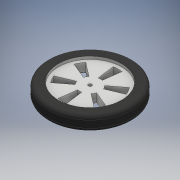
# Autodesk Inventor part: 12 in Wheel
Saved by Autodesk Inventor 2017 (Build 210142000, 142)
## iProperties
Created: 2019-11-18
Part Number: 12 in Wheel
Material: Generic
Document SubType Name: Modeling
Designer: Dell
Density: 1 g/cm^3
Appearance: Default
Author: Dell
Autodesk Inventor part; units mm, degrees
ref_plane "YZ Plane" through (0, 0, 0) normal (1, 0, 0) x (0, 1, 0)
ref_plane "XZ Plane" through (0, 0, 0) normal (0, 1, 0) x (-1, 0, 0)
ref_plane "XY Plane" through (0, 0, 0) normal (0, 0, 1) x (1, 0, 0)
sketch "Sketch1" plane through (0, 0, 0) normal (0, 0, 1) x (1, 0, 0)
  circle A0 centre (0, 0) radius 152.4
  circle A1 centre (0, 0) radius 6.35
  dimension "d0" = 304.8
  dimension "d1" = 12.7
  constraints: 2 centre point, 2 coincident
  measures "d0" diameter of A0
  measures "d1" diameter of A1
extrude "Extrusion1" add sketch "Sketch1" along normal blind 50.8
sketch "Sketch2" plane through (0, 0, 50.8) normal (0, 0, 1) x (1, 0, 0)
  circle A0 centre (0, 0) radius 6.35 projected
  circle A1 centre (0, 0) radius 38.1 construction
  circle A2 centre (0, 0) radius 101.6 construction
  line L0 (7.5, -37.3545) -> (15.7954, -100.3647)
  line L1 (-7.5, -37.3545) -> (-15.7954, -100.3647)
  line L2 (7.5, -37.3545) -> (-7.5, -37.3545) construction
  arc A3 (-15.7954, -100.3647) -> (15.7954, -100.3647) centre (0, 0) ccw
  arc A4 (-7.5, -37.3545) -> (7.5, -37.3545) centre (0, 0) ccw
  circle A5 centre (0, 0) radius 38.1 construction
  circle A6 centre (0, 0) radius 101.6 construction
  line L3 (36.1, -12.1821) -> (94.8161, -36.5031)
  line L4 (28.6, -25.1724) -> (79.0206, -63.8616)
  line L5 (36.1, -12.1821) -> (28.6, -25.1724) construction
  arc A7 (79.0206, -63.8616) -> (94.8161, -36.5031) centre (0, 0) ccw
  arc A8 (28.6, -25.1724) -> (36.1, -12.1821) centre (0, 0) ccw
  circle A9 centre (0, 0) radius 38.1 construction
  circle A10 centre (0, 0) radius 101.6 construction
  line L6 (28.6, 25.1724) -> (79.0206, 63.8616)
  line L7 (36.1, 12.1821) -> (94.8161, 36.5031)
  line L8 (28.6, 25.1724) -> (36.1, 12.1821) construction
  arc A11 (94.8161, 36.5031) -> (79.0206, 63.8616) centre (0, 0) ccw
  arc A12 (36.1, 12.1821) -> (28.6, 25.1724) centre (0, 0) ccw
  circle A13 centre (0, 0) radius 38.1 construction
  circle A14 centre (0, 0) radius 101.6 construction
  line L9 (-7.5, 37.3545) -> (-15.7954, 100.3647)
  line L10 (7.5, 37.3545) -> (15.7954, 100.3647)
  line L11 (-7.5, 37.3545) -> (7.5, 37.3545) construction
  arc A15 (15.7954, 100.3647) -> (-15.7954, 100.3647) centre (0, 0) ccw
  arc A16 (7.5, 37.3545) -> (-7.5, 37.3545) centre (0, 0) ccw
  circle A17 centre (0, 0) radius 38.1 construction
  circle A18 centre (0, 0) radius 101.6 construction
  line L12 (-36.1, 12.1821) -> (-94.8161, 36.5031)
  line L13 (-28.6, 25.1724) -> (-79.0206, 63.8616)
  line L14 (-36.1, 12.1821) -> (-28.6, 25.1724) construction
  arc A19 (-79.0206, 63.8616) -> (-94.8161, 36.5031) centre (0, 0) ccw
  arc A20 (-28.6, 25.1724) -> (-36.1, 12.1821) centre (0, 0) ccw
  circle A21 centre (0, 0) radius 38.1 construction
  circle A22 centre (0, 0) radius 101.6 construction
  line L15 (-28.6, -25.1724) -> (-79.0206, -63.8616)
  line L16 (-36.1, -12.1821) -> (-94.8161, -36.5031)
  line L17 (-28.6, -25.1724) -> (-36.1, -12.1821) construction
  arc A23 (-94.8161, -36.5031) -> (-79.0206, -63.8616) centre (0, 0) ccw
  arc A24 (-36.1, -12.1821) -> (-28.6, -25.1724) centre (0, 0) ccw
  point P0 (0, -37.3545)
  point P1 (0, -101.6)
  point P2 (32.35, -18.6773)
  point P3 (87.9882, -50.8)
  point P4 (32.35, 18.6773)
  point P5 (87.9882, 50.8)
  point P6 (0, 37.3545)
  point P7 (0, 101.6)
  point P8 (-32.35, 18.6773)
  point P9 (-87.9882, 50.8)
  point P10 (-32.35, -18.6773)
  point P11 (-87.9882, -50.8)
  dimension "d4" = 15
  dimension "d5" = 15
  dimension "d6" = 76.2
  dimension "d7" = 203.2
  dimension "d10" = 360
  constraints: 49 point on circle, 36 end point, 24 centre point, 7 coincident, 2 concentric, 2 vertical alignment, 1 horizontal, 1 midpoint, 103 other
  measures "d4" angle of L0 L1
  measures "d5" distance of L0.start L1.start
  measures "d6" diameter of A1
  measures "d7" diameter of A2
extrude "Extrusion2" cut sketch "Sketch2" against normal through all
sketch "Sketch3" plane through (0, 0, 50.8) normal (0, 0, 1) x (1, 0, 0)
  circle A0 centre (0, 0) radius 114.3
  dimension "d14" = 228.6
  constraints: 1 centre point, 1 coincident
  measures "d14" diameter of A0
extrude "Extrusion3" cut sketch "Sketch3" against normal blind 10
sketch "Sketch4" plane through (0, 0, 0) normal (0, 0, -1) x (-1, 0, 0)
  circle A0 centre (0, 0) radius 6.35 projected
  circle A1 centre (0, 0) radius 114.3 projected
extrude "Extrusion4" cut sketch "Sketch4" against normal blind 10 contours A0 | A1
fillet "Fillet1" radius 12.7 2 edges at (-152.4, 0, 0) (-152.4, 0, 50.8)
body "Solid1"
